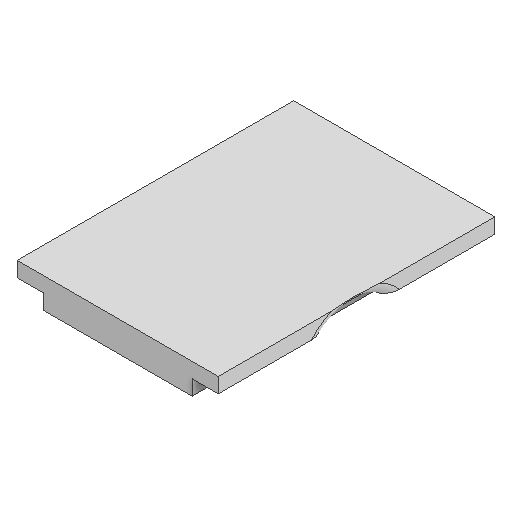
# Autodesk Inventor part: motor cover1
Saved by Autodesk Inventor 2025.3 (Build 293356030, 356C)
## iProperties
Created: 2025-10-25
Part Number: motor cover1
Material: 일반
Document SubType Name: Modeling
Designer: joseph
Density: 1 g/cm^3
Appearance: 기본값
Author: joseph
Autodesk Inventor part; units mm, degrees
ref_plane "YZ Plane" through (0, 0, 0) normal (1, 0, 0) x (0, 1, 0)
ref_plane "XZ Plane" through (0, 0, 0) normal (0, 1, 0) x (-1, 0, 0)
ref_plane "XY Plane" through (0, 0, 0) normal (0, 0, 1) x (1, 0, 0)
sketch "스케치1" plane through (0, 0, 0) normal (0, 1, 0) x (-1, 0, 0)
  line L0 (0, 0) -> (29.6, 0)
  line L1 (29.6, 0) -> (29.6, -55)
  line L2 (29.6, -55) -> (0, -55)
  line L3 (0, -55) -> (0, 0)
  dimension "d0" = 29.6
  dimension "d1" = 55
  constraints: 8 end point, 2 parallel, 1 horizontal, 1 perpendicular
  measures "d0" distance of L1.end L2.end
  measures "d1" distance of L0.end L1.end
extrude "돌출1" add sketch "스케치1" along normal blind 3
sketch "스케치2" plane through (0, 3, 0) normal (0, 1, 0) x (1, 0, 0)
  line L0 (0, 55) -> (-29.6, 55) projected
  line L1 (-29.6, 55) -> (-29.6, 0) projected
  line L2 (-29.6, 0) -> (0, 0) projected
  line L3 (0, 0) -> (0, 55) projected
  line L4 (5.2, 0) -> (-34.8, 0)
  line L5 (-34.8, 0) -> (-34.8, 55)
  line L6 (-34.8, 55) -> (5.2, 55)
  line L7 (5.2, 55) -> (5.2, 0)
  line L8 (0, 55) -> (-29.6, 55) projected
  point P0 (-14.8, 0)
  point P1 (0, 55)
  point P2 (-29.6, 55)
  dimension "d4" = 40
  dimension "d5" = 20
  constraints: 8 end point, 2 parallel, 1 collinear, 1 horizontal, 1 midpoint, 1 perpendicular
  measures "d4" distance of L5.end L6.end
  measures "d5" distance from line of point (-14.8, 0) L5
extrude "돌출2" add sketch "스케치2" along normal blind 3
sketch "스케치3" plane through (5.2, 3, 0) normal (1, 0, 0) x (0, 0, -1)
  line L0 (0, 0) -> (55, 0) projected
  line L1 (55, 0) -> (55, 3) projected
  line L2 (0, 3) -> (55, 3) projected
  line L3 (0, 0) -> (0, 3) projected
  circle A0 centre (27.3, -7.4568) radius 9.5
  point P0 (0, -3)
  point P1 (33.1861, 0)
  point P2 (21.4139, 0)
  dimension "d8" = 19
  constraints: 1 centre point
  measures "d8" diameter of A0
extrude "돌출3" cut sketch "스케치3" against normal blind 3 contours A0 L0 picked at (27.9995, 0.6028)
fillet "모깎기1" radius 2 1 edges at (5.2, 5.0432, -27.3)
